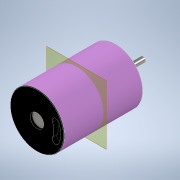
# Autodesk Inventor part: motor
Saved by Autodesk Inventor 2022 (Build 260153000, 153)
## iProperties
Created: 2022-11-23
Part Number: motor
Material: Generisch
Document SubType Name: Modeling
Designer: Friedrich Walmrath
Density: 1 g/cm^3
Appearance: Vorgabe
Author: Friedrich Walmrath
Autodesk Inventor part; units mm, degrees
ref_plane "YZ Plane" through (0, 0, 0) normal (1, 0, 0) x (0, 1, 0)
ref_plane "XZ Plane" through (0, 0, 0) normal (0, 1, 0) x (-1, 0, 0)
ref_plane "XY Plane" through (0, 0, 0) normal (0, 0, 1) x (1, 0, 0)
sketch "Skizze1" plane through (0, 0, 0) normal (0, 0, 1) x (1, 0, 0)
  circle A0 centre (0, 0) radius 12
  dimension "d0" = 24
  constraints: 1 centre point, 1 coincident
  measures "d0" diameter of A0
extrude "Extrusion1" add sketch "Skizze1" along normal blind 35
chamfer "Fase1" distance 0.2 angle 45 2 edges at (-12, 0, 35) (-12, 0, 0)
sketch "Skizze2" plane through (0, 0, 0) normal (0, 0, -1) x (-1, 0, 0)
  circle A0 centre (0, 0) radius 3
  dimension "d7" = 6
  constraints: 1 centre point, 1 coincident
  measures "d7" diameter of A0
extrude "Extrusion2" cut sketch "Skizze2" against normal blind 1
ref_plane "Arbeitsebene1" through (0, 0, 17.5) normal (0, 0, -1) x (-1, 0, 0)
mirror "Spiegeln1" about plane through (0, 0, 17.5) normal (0, 0, -1) of "Extrusion2"
sketch "Skizze3" plane through (0, 0, 1) normal (0, 0, -1) x (-1, 0, 0)
  circle A0 centre (0, 0) radius 1.5
  dimension "d10" = 3
  constraints: 1 centre point, 1 coincident
  measures "d10" diameter of A0
extrude "Extrusion3" add sketch "Skizze3" along normal blind 1
sketch "Skizze4" plane through (0, 0, 0) normal (0, 0, -1) x (-1, 0, 0)
  circle A0 centre (0, 0) radius 1.15
  dimension "d13" = 2.3
  constraints: 1 centre point, 1 coincident
  measures "d13" diameter of A0
extrude "Extrusion4" add sketch "Skizze4" along normal blind 12
sketch "Skizze5" plane through (0, 0, -12) normal (0, 0, -1) x (-1, 0, 0)
  circle A0 centre (0, 0) radius 1.15 projected
  line L0 (0.85, 0.7746) -> (0.85, -0.7746)
  line L1 (0.85, 0) -> (-1.15, 0) construction
  dimension "d16" = 2
  constraints: 4 end point, 3 point on circle, 1 horizontal, 1 midpoint, 1 vertical
  measures "d16" distance of L1.start L1.end
extrude "Extrusion5" cut sketch "Skizze5" against normal blind 10 contours A0 L0 picked at (0.9044, -0.1813)
sketch "Skizze6" plane through (0, 0, 35) normal (0, 0, 1) x (1, 0, 0)
  circle A0 centre (0, 0) radius 3 projected
  arc A1 (8.2916, -3.5) -> (8.2916, 3.5) centre (0, 0) ccw construction
  arc A2 (9.6735, -4.0833) -> (9.6735, 4.0833) centre (0, 0) ccw
  arc A3 (6.9096, -2.9167) -> (6.9096, 2.9167) centre (0, 0) ccw
  arc A4 (6.9096, -2.9167) -> (9.6735, -4.0833) centre (8.2916, -3.5) ccw
  arc A5 (9.6735, 4.0833) -> (6.9096, 2.9167) centre (8.2916, 3.5) ccw
  dimension "d19" = 1.5
  dimension "d20" = 7
  dimension "d21" = 3.5
  dimension "d22" = 9
  constraints: 10 point on circle, 5 centre point, 4 tangent, 1 coincident
  measures "d19" radius of A4
  measures "d20" distance of A1.end A1.start
  measures "d21" vertical distance of point (0, 0) A1.start
  measures "d22" radius of A1
extrude "Extrusion6" cut sketch "Skizze6" against normal blind 2 contours A4 A3 A5 A2
sketch "Skizze7" plane through (0, 0, 0) normal (0, 0, -1) x (-1, 0, 0)
  circle A0 centre (0, 8.5) radius 1.5
  point P0 (0, 0)
  dimension "d25" = 3
  dimension "d26" = 8.5
  constraints: 1 centre point, 1 vertical alignment
  measures "d25" diameter of A0
  measures "d26" distance of point (0, 0) A0.centre
extrude "Extrusion7" cut sketch "Skizze7" against normal blind 5
thread "Gewinde1" size "M3x0.5" class "6H" standard "ANSI Metric M Profile" full length
chamfer "Fase2" distance 0.3 angle 45 1 edges at (1.5, 8.5, 0)
pattern_circular "Runde Anordnung1" count 6 over 360 about axis through (0, 0, 0) along (0, 0, -1) of "Extrusion7", "Fase2"
ref_plane "Arbeitsebene2" through (0, 0, 17.5) normal (0, 0, -1) x (-1, 0, 0)
